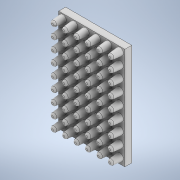
# Autodesk Inventor part: Mold_equalSpacing_2mm
Saved by Autodesk Inventor 2021 (Build 250183000, 183)
## iProperties
Created: 2021-04-08
Part Number: Mold_equalSpacing_2mm
Material: Generic
Document SubType Name: Modeling
Designer: Olivi
Density: 1 g/cm^3
Appearance: Default
Author: Olivi
Autodesk Inventor part; units mm, degrees
ref_plane "YZ Plane" through (0, 0, 0) normal (1, 0, 0) x (0, 1, 0)
ref_plane "XZ Plane" through (0, 0, 0) normal (0, 1, 0) x (-1, 0, 0)
ref_plane "XY Plane" through (0, 0, 0) normal (0, 0, 1) x (1, 0, 0)
sketch "Sketch1" plane through (0, 0, 0) normal (0, 0, 1) x (1, 0, 0)
  line L0 (0, 0) -> (19.1, 0)
  line L1 (19.1, 0) -> (19.1, 29.4)
  line L2 (19.1, 29.4) -> (0, 29.4)
  line L3 (0, 29.4) -> (0, 0)
  dimension "d0" = 19.1
  dimension "d1" = 29.4
  constraints: 8 end point, 2 horizontal, 2 perpendicular
  measures "d0" distance of L0.start L0.end
  measures "d1" distance of L0.end L1.end
extrude "Extrusion1" add sketch "Sketch1" along normal blind 2
sketch "Sketch2" plane through (0, 0, 2) normal (0, 0, 1) x (1, 0, 0)
  line L0 (0, 29.4) -> (0, 0) projected
  circle A0 centre (1.2, 28.2) radius 1
  line L1 (19.1, 29.4) -> (0, 29.4) projected
  dimension "d6" = 2
  dimension "d7" = 1.2
  dimension "d8" = 1.2
  constraints: 1 centre point
  measures "d6" diameter of A0
  measures "d7" distance from line of L0 A0.centre
  measures "d8" distance from line of L1 A0.centre
ref_plane "Work Plane1" through (0, 0, 5) normal (0, 0, 1) x (1, 0, 0)
ref_plane "Work Plane2" through (0, 0, 4.5) normal (0, 0, 1) x (1, 0, 0)
extrude "Extrusion3" add sketch "Sketch2" along normal blind 3 draft -5
pattern_linear "Rectangular Pattern1" count 6 spacing 3.3 along (1, 0, 0) count 9 spacing 3.3 along (0, -1, 0) of "Extrusion3"
fillet "Fillet1" radius 0.5 1 edges at (0.4625, 28.2, 5) curvature continuous yes
fillet "Fillet2" radius 0.5 53 edges at (3.7625, 28.2, 5) (7.0625, 28.2, 5) (10.3625, 28.2, 5) (13.6625, 28.2, 5) (16.9625, 28.2, 5) (0.4625, 24.9, 5) (3.7625, 24.9, 5) (7.0625, 24.9, 5) (10.3625, 24.9, 5) (13.6625, 24.9, 5) (16.9625, 24.9, 5) (0.4625, 21.6, 5) (3.7625, 21.6, 5) (7.0625, 21.6, 5) (10.3625, 21.6, 5) (13.6625, 21.6, 5) (16.9625, 21.6, 5) (0.4625, 18.3, 5) (3.7625, 18.3, 5) (7.0625, 18.3, 5) (10.3625, 18.3, 5) (13.6625, 18.3, 5) (16.9625, 18.3, 5) (0.4625, 15, 5) (3.7625, 15, 5) (7.0625, 15, 5) (10.3625, 15, 5) (13.6625, 15, 5) (16.9625, 15, 5) (0.4625, 11.7, 5) (3.7625, 11.7, 5) (7.0625, 11.7, 5) (10.3625, 11.7, 5) (13.6625, 11.7, 5) (16.9625, 11.7, 5) (0.4625, 8.4, 5) (3.7625, 8.4, 5) (7.0625, 8.4, 5) (10.3625, 8.4, 5) (13.6625, 8.4, 5) (16.9625, 8.4, 5) (0.4625, 5.1, 5) (3.7625, 5.1, 5) (7.0625, 5.1, 5) (10.3625, 5.1, 5) (13.6625, 5.1, 5) (16.9625, 5.1, 5) (0.4625, 1.8, 5) (3.7625, 1.8, 5) (7.0625, 1.8, 5) (10.3625, 1.8, 5) (13.6625, 1.8, 5) (16.9625, 1.8, 5)
body "Solid1"
